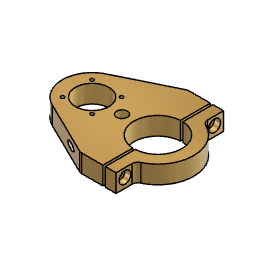
BC linear drive top bearing fixture v5 (Autodesk Fusion 360 design; units mm, degrees)
Autodesk Fusion 360 part; units mm, degrees
note: some values were not read from the file. Set by a fixed rule: the direction of a hole.
sketch "Sketch1" plane through (0, 0, 0) normal (0, 1, 0) x (1, 0, 0)
  circle A0 centre (0, 0) radius 17.5 construction
  line L0 (-12.3744, 12.3744) -> (12.3744, 12.3744) construction
  line L1 (12.3744, 12.3744) -> (12.3744, -12.3744) construction
  line L2 (12.3744, -12.3744) -> (-12.3744, -12.3744) construction
  line L3 (-12.3744, -12.3744) -> (-12.3744, 12.3744) construction
  circle A1 centre (0, 0) radius 14
  circle A2 centre (55, 0) radius 20
  line L4 (65, 28.2843) -> (65, 45)
  line L5 (65, 45) -> (35, 45)
  line L6 (35, 45) -> (-11.0043, 22.4478)
  arc A3 (-11.0043, 22.4478) -> (-25, 0) centre (0, 0) ccw
  arc A4 (85, 0) -> (65, 28.2843) centre (55, 0) ccw
  line L7 (1.75, 0) -> (22.5, 0)
  arc A5 (65, -28.2843) -> (85, 0) centre (55, 0) ccw
  line L8 (65, -28.2843) -> (65, -45)
  line L9 (65, -45) -> (35, -45)
  line L10 (35, -45) -> (-11.0043, -22.4478)
  arc A6 (-25, 0) -> (-11.0043, -22.4478) centre (0, 0) ccw
  point P0 (25, 0)
  dimension "d1" = 35
  dimension "d2" = 28
  dimension "d3" = 40
  dimension "d4" = 55
  dimension "d5" = 25
  dimension "d6" = 30
  dimension "d7" = 10
  dimension "d8" = 30
  dimension "d9" = 45
  dimension "d31" = 30
  constraint coincident A0.centre A1.centre
  constraint horizontal L0
  constraint vertical L1
  constraint horizontal L2
  constraint vertical L3
  constraint coincident A0 L1.end
  constraint coincident A0 L0.start
  constraint equal L0 L1
  constraint coincident A0 L0.end
  constraint concentric A0 A1
  constraint horizontal A0.centre A2.centre
  constraint vertical L4
  constraint perpendicular L4 L5
  constraint tangent L6 A3
  constraint coincident A2.centre A4.centre
  constraint horizontal A2.centre A4.start
  constraint horizontal A0.centre A3.end
  constraint symmetric L4.start L7 A5.start
  constraint symmetric L4.end L7 L8.end
  constraint symmetric L5.end L7 L9.end
  constraint symmetric L6.end L7 L10.end
  constraint symmetric A3.end L7 A6.start
  constraint symmetric A3 L7 A6
  constraint symmetric A4.start L7 A5.end
  constraint symmetric A4 L7 A5
  constraint horizontal A2.centre P0
  measures "d1" diameter of A0
  measures "d2" diameter of A1
  measures "d3" diameter of A2
  measures "d4" distance of A0.centre A2.centre
  measures "d5" radius of A3
  measures "d6" radius of A4
  measures "d7" distance of A2.centre L4
  measures "d8" distance of L4.end L5.end
  measures "d9" distance of A2.centre L5
  measures "d31" distance of A2.centre P0
extrude "Extrude1" add sketch "Sketch1" along normal blind 15 makes body 1
hole "Hole1" at (-12.3744, 0, 12.3744) at (12.3744, 0, 12.3744) at (12.3744, 0, -12.3744) at (-12.3744, 0, -12.3744) direction (0, 1, 0) diameter 2.93 end through all bodies 1
thread "Thread2" "ISO Metric profile 3.5 M3.5x0.6 6H" thread offset 0 thread depth 10
ref_plane "WorkPlane1" through (55, 0, 0) normal (1, 0, 0) x (0, 1, 0)
sketch "Sketch2" plane through (55, 0, 0) normal (1, 0, 0) x (0, 0, -1)
  line L0 (-52.531, 37.047) -> (45, 37.047)
  line L1 (45, 37.047) -> (45, -15)
  line L2 (45, -15) -> (-52.531, -15)
  line L3 (-52.531, -15) -> (-52.531, 37.047)
  constraint horizontal L0
  constraint vertical L1
  constraint horizontal L2
  constraint vertical L3
extrude "Extrude2" cut sketch "Sketch2" along normal mid plane 2 bodies 1 makes body 2 at (73.8112, 10, -23.3696)
sketch "Sketch3" plane through (65, 0, 0) normal (1, 0, 0) x (0, 0, -1)
  line L0 (28.2843, 0) -> (45, 0)
  line L1 (45, 0) -> (45, 15)
  line L2 (45, 15) -> (28.2843, 15)
  line L3 (28.2843, 15) -> (28.2843, 0)
  point P0 (37.5, 8)
  dimension "d23" = 7.5
  measures "d23" distance of L1 P0
hole "Hole2" at (65, 8, -37.5) direction (-1, 0, 0) diameter 5.5 depth 10 tip angle 180 counterbore diameter 10 counterbore depth 5 bodies 2
hole "Hole3" at (65, 8, -37.5) direction (-1, 0, 0) diameter 5.029 end through all bodies 1
thread "Thread1" "ISO Metric profile 5.5 M5.5x0.5 6H" thread offset 0 thread depth 10
mirror "Mirror1" about plane through (0, 0, 0) normal (0, 0, 1) of "Hole2", "Hole3"
fillet "Fillet1" radius 5 4 edges at (35, 7.5, -45) (35, 7.5, 45) (65, 7.5, -28.2843) (65, 7.5, 28.2843) on bodies 1 2
hole "Hole4" at (25, 0, 0) direction (0, 1, 0) diameter 9 end through all bodies 1
copy_body "Body->Comp1" bodies 1 removing the originals makes body 3 in component "console"
copy_body "Body->Comp2" bodies 2 removing the originals makes body 4 in component "brace"
component "console" placed x (1, 0, 0) y (0, 1, 0) z (0, 0, 1) at (0, 0, 0)
component "brace" placed x (1, 0, 0) y (0, 1, 0) z (0, 0, 1) at (0, 0, 0)
named bodies: "console", "brace"
